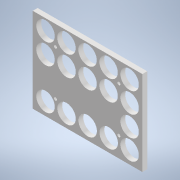
# Autodesk Inventor part: Conectores1
Saved by Autodesk Inventor 2020.3 (Build 243373000, 373)
## iProperties
Created: 2021-04-09
Part Number: Conectores1
Material: Generic
Document SubType Name: Modeling
Designer: juanp
Density: 1 g/cm^3
Appearance: Default
Autodesk Inventor part; units mm, degrees
(part 1 of 8)
ref_plane "YZ Plane" through (0, 0, 0) normal (1, 0, 0) x (0, 1, 0)
ref_plane "XZ Plane" through (0, 0, 0) normal (0, 1, 0) x (-1, 0, 0)
ref_plane "XY Plane" through (0, 0, 0) normal (0, 0, 1) x (1, 0, 0)
sketch "Sketch1" plane through (0, 0, 0) normal (0, 0, 1) x (1, 0, 0)
  arc A0 (61.2864, 36.699) -> (61.2864, 35.945) centre (61.2864, 36.322) ccw
  arc A1 (61.2864, 35.945) -> (61.2864, 36.699) centre (61.2864, 36.322) ccw
  arc A2 (61.2864, 36.699) -> (61.2864, 35.945) centre (61.2864, 36.322) ccw
  arc A3 (61.2864, 35.945) -> (61.2864, 36.699) centre (61.2864, 36.322) ccw
  arc A4 (61.2864, 34.159) -> (61.2864, 33.405) centre (61.2864, 33.782) ccw
  arc A5 (61.2864, 33.405) -> (61.2864, 34.159) centre (61.2864, 33.782) ccw
  arc A6 (61.2864, 34.159) -> (61.2864, 33.405) centre (61.2864, 33.782) ccw
  arc A7 (61.2864, 33.405) -> (61.2864, 34.159) centre (61.2864, 33.782) ccw
  arc A8 (58.7464, 36.699) -> (58.7464, 35.945) centre (58.7464, 36.322) ccw
  arc A9 (58.7464, 35.945) -> (58.7464, 36.699) centre (58.7464, 36.322) ccw
  arc A10 (58.7464, 36.699) -> (58.7464, 35.945) centre (58.7464, 36.322) ccw
  arc A11 (58.7464, 35.945) -> (58.7464, 36.699) centre (58.7464, 36.322) ccw
  arc A12 (58.7464, 34.159) -> (58.7464, 33.405) centre (58.7464, 33.782) ccw
  arc A13 (58.7464, 33.405) -> (58.7464, 34.159) centre (58.7464, 33.782) ccw
  arc A14 (58.7464, 34.159) -> (58.7464, 33.405) centre (58.7464, 33.782) ccw
  arc A15 (58.7464, 33.405) -> (58.7464, 34.159) centre (58.7464, 33.782) ccw
  arc A16 (56.2064, 36.699) -> (56.2064, 35.945) centre (56.2064, 36.322) ccw
  arc A17 (56.2064, 35.945) -> (56.2064, 36.699) centre (56.2064, 36.322) ccw
  arc A18 (56.2064, 36.699) -> (56.2064, 35.945) centre (56.2064, 36.322) ccw
  arc A19 (56.2064, 35.945) -> (56.2064, 36.699) centre (56.2064, 36.322) ccw
  arc A20 (56.2064, 34.159) -> (56.2064, 33.405) centre (56.2064, 33.782) ccw
  arc A21 (56.2064, 33.405) -> (56.2064, 34.159) centre (56.2064, 33.782) ccw
  arc A22 (56.2064, 34.159) -> (56.2064, 33.405) centre (56.2064, 33.782) ccw
  arc A23 (56.2064, 33.405) -> (56.2064, 34.159) centre (56.2064, 33.782) ccw
  arc A24 (53.6664, 36.699) -> (53.6664, 35.945) centre (53.6664, 36.322) ccw
  arc A25 (53.6664, 35.945) -> (53.6664, 36.699) centre (53.6664, 36.322) ccw
  arc A26 (53.6664, 36.699) -> (53.6664, 35.945) centre (53.6664, 36.322) ccw
  arc A27 (53.6664, 35.945) -> (53.6664, 36.699) centre (53.6664, 36.322) ccw
  arc A28 (53.6664, 34.159) -> (53.6664, 33.405) centre (53.6664, 33.782) ccw
  arc A29 (53.6664, 33.405) -> (53.6664, 34.159) centre (53.6664, 33.782) ccw
  arc A30 (53.6664, 34.159) -> (53.6664, 33.405) centre (53.6664, 33.782) ccw
  arc A31 (53.6664, 33.405) -> (53.6664, 34.159) centre (53.6664, 33.782) ccw
  arc A32 (51.1264, 36.699) -> (51.1264, 35.945) centre (51.1264, 36.322) ccw
  arc A33 (51.1264, 35.945) -> (51.1264, 36.699) centre (51.1264, 36.322) ccw
  arc A34 (51.1264, 36.699) -> (51.1264, 35.945) centre (51.1264, 36.322) ccw
  arc A35 (51.1264, 35.945) -> (51.1264, 36.699) centre (51.1264, 36.322) ccw
  arc A36 (51.1264, 34.159) -> (51.1264, 33.405) centre (51.1264, 33.782) ccw
  arc A37 (51.1264, 33.405) -> (51.1264, 34.159) centre (51.1264, 33.782) ccw
  arc A38 (51.1264, 34.159) -> (51.1264, 33.405) centre (51.1264, 33.782) ccw
  arc A39 (51.1264, 33.405) -> (51.1264, 34.159) centre (51.1264, 33.782) ccw
  arc A40 (9.0927, 77.8361) -> (9.0927, 75.8281) centre (9.0927, 76.8321) ccw
  arc A41 (9.0927, 75.8281) -> (9.0927, 77.8361) centre (9.0927, 76.8321) ccw
  arc A42 (9.0927, 77.8361) -> (9.0927, 75.8281) centre (9.0927, 76.8321) ccw
  arc A43 (9.0927, 75.8281) -> (9.0927, 77.8361) centre (9.0927, 76.8321) ccw
  arc A44 (12.0927, 72.8361) -> (12.0927, 70.8281) centre (12.0927, 71.8321) ccw
  arc A45 (12.0927, 70.8281) -> (12.0927, 72.8361) centre (12.0927, 71.8321) ccw
  arc A46 (12.0927, 72.8361) -> (12.0927, 70.8281) centre (12.0927, 71.8321) ccw
  arc A47 (12.0927, 70.8281) -> (12.0927, 72.8361) centre (12.0927, 71.8321) ccw
  arc A48 (15.0927, 77.8361) -> (15.0927, 75.8281) centre (15.0927, 76.8321) ccw
  arc A49 (15.0927, 75.8281) -> (15.0927, 77.8361) centre (15.0927, 76.8321) ccw
  arc A50 (15.0927, 77.8361) -> (15.0927, 75.8281) centre (15.0927, 76.8321) ccw
  arc A51 (15.0927, 75.8281) -> (15.0927, 77.8361) centre (15.0927, 76.8321) ccw
  arc A52 (101.4424, 52.9529) -> (101.4424, 54.9609) centre (101.4424, 53.9569) ccw
  arc A53 (101.4424, 54.9609) -> (101.4424, 52.9529) centre (101.4424, 53.9569) ccw
  arc A54 (101.4424, 52.9529) -> (101.4424, 54.9609) centre (101.4424, 53.9569) ccw
  arc A55 (101.4424, 54.9609) -> (101.4424, 52.9529) centre (101.4424, 53.9569) ccw
  arc A56 (95.4424, 52.9529) -> (95.4424, 54.9609) centre (95.4424, 53.9569) ccw
  arc A57 (95.4424, 54.9609) -> (95.4424, 52.9529) centre (95.4424, 53.9569) ccw
  arc A58 (95.4424, 52.9529) -> (95.4424, 54.9609) centre (95.4424, 53.9569) ccw
  arc A59 (95.4424, 54.9609) -> (95.4424, 52.9529) centre (95.4424, 53.9569) ccw
  line L0 (77.9954, 35.7425) -> (76.9954, 35.7425)
  line L1 (76.9954, 35.7425) -> (76.9954, 34.7425)
  line L2 (76.9954, 34.7425) -> (77.9954, 34.7425)
  line L3 (77.9954, 34.7425) -> (77.9954, 35.7425)
  line L4 (80.01, 36.2331) -> (80.01, 34.2519)
  arc A60 (79.5147, 34.2519) -> (80.5053, 34.2519) centre (80.01, 34.2519) ccw
  arc A61 (80.5053, 36.2331) -> (79.5147, 36.2331) centre (80.01, 36.2331) ccw
  line L5 (80.01, 36.2331) -> (80.01, 34.2519)
  arc A62 (79.5147, 34.2519) -> (80.5053, 34.2519) centre (80.01, 34.2519) ccw
  arc A63 (80.5053, 36.2331) -> (79.5147, 36.2331) centre (80.01, 36.2331) ccw
  line L6 (74.9808, 36.2331) -> (74.9808, 34.2519)
  arc A64 (74.4855, 34.2519) -> (75.4761, 34.2519) centre (74.9808, 34.2519) ccw
  arc A65 (75.4761, 36.2331) -> (74.4855, 36.2331) centre (74.9808, 36.2331) ccw
  line L7 (74.9808, 36.2331) -> (74.9808, 34.2519)
  arc A66 (74.4855, 34.2519) -> (75.4761, 34.2519) centre (74.9808, 34.2519) ccw
  arc A67 (75.4761, 36.2331) -> (74.4855, 36.2331) centre (74.9808, 36.2331) ccw
  arc A68 (35.56, 36.699) -> (35.56, 35.945) centre (35.56, 36.322) ccw
  arc A69 (35.56, 35.945) -> (35.56, 36.699) centre (35.56, 36.322) ccw
  arc A70 (35.56, 36.699) -> (35.56, 35.945) centre (35.56, 36.322) ccw
  arc A71 (35.56, 35.945) -> (35.56, 36.699) centre (35.56, 36.322) ccw
  arc A72 (35.56, 34.159) -> (35.56, 33.405) centre (35.56, 33.782) ccw
  arc A73 (35.56, 33.405) -> (35.56, 34.159) centre (35.56, 33.782) ccw
  arc A74 (35.56, 34.159) -> (35.56, 33.405) centre (35.56, 33.782) ccw
  arc A75 (35.56, 33.405) -> (35.56, 34.159) centre (35.56, 33.782) ccw
  arc A76 (33.02, 36.699) -> (33.02, 35.945) centre (33.02, 36.322) ccw
  arc A77 (33.02, 35.945) -> (33.02, 36.699) centre (33.02, 36.322) ccw
  arc A78 (33.02, 36.699) -> (33.02, 35.945) centre (33.02, 36.322) ccw
  arc A79 (33.02, 35.945) -> (33.02, 36.699) centre (33.02, 36.322) ccw
  arc A80 (33.02, 34.159) -> (33.02, 33.405) centre (33.02, 33.782) ccw
  arc A81 (33.02, 33.405) -> (33.02, 34.159) centre (33.02, 33.782) ccw
  arc A82 (33.02, 34.159) -> (33.02, 33.405) centre (33.02, 33.782) ccw
  arc A83 (33.02, 33.405) -> (33.02, 34.159) centre (33.02, 33.782) ccw
  arc A84 (30.48, 36.699) -> (30.48, 35.945) centre (30.48, 36.322) ccw
  arc A85 (30.48, 35.945) -> (30.48, 36.699) centre (30.48, 36.322) ccw
  arc A86 (30.48, 36.699) -> (30.48, 35.945) centre (30.48, 36.322) ccw
  arc A87 (30.48, 35.945) -> (30.48, 36.699) centre (30.48, 36.322) ccw
  arc A88 (30.48, 34.159) -> (30.48, 33.405) centre (30.48, 33.782) ccw
  arc A89 (30.48, 33.405) -> (30.48, 34.159) centre (30.48, 33.782) ccw
  arc A90 (30.48, 34.159) -> (30.48, 33.405) centre (30.48, 33.782) ccw
  arc A91 (30.48, 33.405) -> (30.48, 34.159) centre (30.48, 33.782) ccw
  arc A92 (27.94, 36.699) -> (27.94, 35.945) centre (27.94, 36.322) ccw
  arc A93 (27.94, 35.945) -> (27.94, 36.699) centre (27.94, 36.322) ccw
  arc A94 (27.94, 36.699) -> (27.94, 35.945) centre (27.94, 36.322) ccw
  arc A95 (27.94, 35.945) -> (27.94, 36.699) centre (27.94, 36.322) ccw
  arc A96 (27.94, 34.159) -> (27.94, 33.405) centre (27.94, 33.782) ccw
  arc A97 (27.94, 33.405) -> (27.94, 34.159) centre (27.94, 33.782) ccw
  arc A98 (27.94, 34.159) -> (27.94, 33.405) centre (27.94, 33.782) ccw
  arc A99 (27.94, 33.405) -> (27.94, 34.159) centre (27.94, 33.782) ccw
  arc A100 (25.4, 36.699) -> (25.4, 35.945) centre (25.4, 36.322) ccw
  arc A101 (25.4, 35.945) -> (25.4, 36.699) centre (25.4, 36.322) ccw
  arc A102 (25.4, 36.699) -> (25.4, 35.945) centre (25.4, 36.322) ccw
  arc A103 (25.4, 35.945) -> (25.4, 36.699) centre (25.4, 36.322) ccw
  arc A104 (25.4, 34.159) -> (25.4, 33.405) centre (25.4, 33.782) ccw
  arc A105 (25.4, 33.405) -> (25.4, 34.159) centre (25.4, 33.782) ccw
  arc A106 (25.4, 34.159) -> (25.4, 33.405) centre (25.4, 33.782) ccw
  arc A107 (25.4, 33.405) -> (25.4, 34.159) centre (25.4, 33.782) ccw
  arc A108 (22.86, 36.699) -> (22.86, 35.945) centre (22.86, 36.322) ccw
  arc A109 (22.86, 35.945) -> (22.86, 36.699) centre (22.86, 36.322) ccw
  arc A110 (22.86, 36.699) -> (22.86, 35.945) centre (22.86, 36.322) ccw
  arc A111 (22.86, 35.945) -> (22.86, 36.699) centre (22.86, 36.322) ccw
  arc A112 (22.86, 34.159) -> (22.86, 33.405) centre (22.86, 33.782) ccw
  arc A113 (22.86, 33.405) -> (22.86, 34.159) centre (22.86, 33.782) ccw
  arc A114 (22.86, 34.159) -> (22.86, 33.405) centre (22.86, 33.782) ccw
  arc A115 (22.86, 33.405) -> (22.86, 34.159) centre (22.86, 33.782) ccw
  arc A116 (20.32, 36.699) -> (20.32, 35.945) centre (20.32, 36.322) ccw
  arc A117 (20.32, 35.945) -> (20.32, 36.699) centre (20.32, 36.322) ccw
  arc A118 (20.32, 36.699) -> (20.32, 35.945) centre (20.32, 36.322) ccw
  arc A119 (20.32, 35.945) -> (20.32, 36.699) centre (20.32, 36.322) ccw
  arc A120 (20.32, 34.159) -> (20.32, 33.405) centre (20.32, 33.782) ccw
  arc A121 (20.32, 33.405) -> (20.32, 34.159) centre (20.32, 33.782) ccw
  arc A122 (20.32, 34.159) -> (20.32, 33.405) centre (20.32, 33.782) ccw
  arc A123 (20.32, 33.405) -> (20.32, 34.159) centre (20.32, 33.782) ccw
  arc A124 (17.78, 36.699) -> (17.78, 35.945) centre (17.78, 36.322) ccw
  arc A125 (17.78, 35.945) -> (17.78, 36.699) centre (17.78, 36.322) ccw
  arc A126 (17.78, 36.699) -> (17.78, 35.945) centre (17.78, 36.322) ccw
  arc A127 (17.78, 35.945) -> (17.78, 36.699) centre (17.78, 36.322) ccw
  arc A128 (17.78, 34.159) -> (17.78, 33.405) centre (17.78, 33.782) ccw
  arc A129 (17.78, 33.405) -> (17.78, 34.159) centre (17.78, 33.782) ccw
  arc A130 (17.78, 34.159) -> (17.78, 33.405) centre (17.78, 33.782) ccw
  arc A131 (17.78, 33.405) -> (17.78, 34.159) centre (17.78, 33.782) ccw
  arc A132 (15.24, 36.699) -> (15.24, 35.945) centre (15.24, 36.322) ccw
  arc A133 (15.24, 35.945) -> (15.24, 36.699) centre (15.24, 36.322) ccw
  arc A134 (15.24, 36.699) -> (15.24, 35.945) centre (15.24, 36.322) ccw
  arc A135 (15.24, 35.945) -> (15.24, 36.699) centre (15.24, 36.322) ccw
  arc A136 (15.24, 34.159) -> (15.24, 33.405) centre (15.24, 33.782) ccw
  arc A137 (15.24, 33.405) -> (15.24, 34.159) centre (15.24, 33.782) ccw
  arc A138 (15.24, 34.159) -> (15.24, 33.405) centre (15.24, 33.782) ccw
  arc A139 (15.24, 33.405) -> (15.24, 34.159) centre (15.24, 33.782) ccw
  arc A140 (12.7, 36.699) -> (12.7, 35.945) centre (12.7, 36.322) ccw
  arc A141 (12.7, 35.945) -> (12.7, 36.699) centre (12.7, 36.322) ccw
  arc A142 (12.7, 36.699) -> (12.7, 35.945) centre (12.7, 36.322) ccw
  arc A143 (12.7, 35.945) -> (12.7, 36.699) centre (12.7, 36.322) ccw
  arc A144 (12.7, 34.159) -> (12.7, 33.405) centre (12.7, 33.782) ccw
  arc A145 (12.7, 33.405) -> (12.7, 34.159) centre (12.7, 33.782) ccw
  arc A146 (12.7, 34.159) -> (12.7, 33.405) centre (12.7, 33.782) ccw
  arc A147 (12.7, 33.405) -> (12.7, 34.159) centre (12.7, 33.782) ccw
  arc A148 (10.16, 36.699) -> (10.16, 35.945) centre (10.16, 36.322) ccw
  arc A149 (10.16, 35.945) -> (10.16, 36.699) centre (10.16, 36.322) ccw
  arc A150 (10.16, 36.699) -> (10.16, 35.945) centre (10.16, 36.322) ccw
  arc A151 (10.16, 35.945) -> (10.16, 36.699) centre (10.16, 36.322) ccw
  arc A152 (10.16, 34.159) -> (10.16, 33.405) centre (10.16, 33.782) ccw
  arc A153 (10.16, 33.405) -> (10.16, 34.159) centre (10.16, 33.782) ccw
  arc A154 (10.16, 34.159) -> (10.16, 33.405) centre (10.16, 33.782) ccw
  arc A155 (10.16, 33.405) -> (10.16, 34.159) centre (10.16, 33.782) ccw
  arc A156 (7.62, 36.699) -> (7.62, 35.945) centre (7.62, 36.322) ccw
  arc A157 (7.62, 35.945) -> (7.62, 36.699) centre (7.62, 36.322) ccw
  arc A158 (7.62, 36.699) -> (7.62, 35.945) centre (7.62, 36.322) ccw
  arc A159 (7.62, 35.945) -> (7.62, 36.699) centre (7.62, 36.322) ccw
  arc A160 (7.62, 34.159) -> (7.62, 33.405) centre (7.62, 33.782) ccw
  arc A161 (7.62, 33.405) -> (7.62, 34.159) centre (7.62, 33.782) ccw
  arc A162 (7.62, 34.159) -> (7.62, 33.405) centre (7.62, 33.782) ccw
  arc A163 (7.62, 33.405) -> (7.62, 34.159) centre (7.62, 33.782) ccw
  arc A164 (74.3504, 57.4609) -> (74.3504, 55.4529) centre (74.3504, 56.4569) ccw
  arc A165 (74.3504, 55.4529) -> (74.3504, 57.4609) centre (74.3504, 56.4569) ccw
  arc A166 (74.3504, 57.4609) -> (74.3504, 55.4529) centre (74.3504, 56.4569) ccw
  arc A167 (74.3504, 55.4529) -> (74.3504, 57.4609) centre (74.3504, 56.4569) ccw
  arc A168 (74.3504, 52.4609) -> (74.3504, 50.4529) centre (74.3504, 51.4569) ccw
  arc A169 (74.3504, 50.4529) -> (74.3504, 52.4609) centre (74.3504, 51.4569) ccw
  arc A170 (74.3504, 52.4609) -> (74.3504, 50.4529) centre (74.3504, 51.4569) ccw
  arc A171 (74.3504, 50.4529) -> (74.3504, 52.4609) centre (74.3504, 51.4569) ccw
  arc A172 (79.3504, 52.4609) -> (79.3504, 50.4529) centre (79.3504, 51.4569) ccw
  arc A173 (79.3504, 50.4529) -> (79.3504, 52.4609) centre (79.3504, 51.4569) ccw
  arc A174 (79.3504, 52.4609) -> (79.3504, 50.4529) centre (79.3504, 51.4569) ccw
  arc A175 (79.3504, 50.4529) -> (79.3504, 52.4609) centre (79.3504, 51.4569) ccw
  arc A176 (79.3504, 57.4609) -> (79.3504, 55.4529) centre (79.3504, 56.4569) ccw
  arc A177 (79.3504, 55.4529) -> (79.3504, 57.4609) centre (79.3504, 56.4569) ccw
  arc A178 (79.3504, 57.4609) -> (79.3504, 55.4529) centre (79.3504, 56.4569) ccw
  arc A179 (79.3504, 55.4529) -> (79.3504, 57.4609) centre (79.3504, 56.4569) ccw
  line L8 (23.36, 25.392) -> (22.36, 25.392)
  line L9 (22.36, 25.392) -> (22.36, 24.392)
  line L10 (22.36, 24.392) -> (23.36, 24.392)
  line L11 (23.36, 24.392) -> (23.36, 25.392)
  line L12 (23.36, 26.408) -> (22.36, 26.408)
  line L13 (22.36, 26.408) -> (22.36, 25.408)
  line L14 (22.36, 25.408) -> (23.36, 25.408)
  line L15 (23.36, 25.408) -> (23.36, 26.408)
  line L16 (20.82, 25.392) -> (19.82, 25.392)
  line L17 (19.82, 25.392) -> (19.82, 24.392)
  line L18 (19.82, 24.392) -> (20.82, 24.392)
  line L19 (20.82, 24.392) -> (20.82, 25.392)
  line L20 (20.82, 26.408) -> (19.82, 26.408)
  line L21 (19.82, 26.408) -> (19.82, 25.408)
  line L22 (19.82, 25.408) -> (20.82, 25.408)
  line L23 (20.82, 25.408) -> (20.82, 26.408)
  line L24 (18.28, 25.392) -> (17.28, 25.392)
  line L25 (17.28, 25.392) -> (17.28, 24.392)
  line L26 (17.28, 24.392) -> (18.28, 24.392)
  line L27 (18.28, 24.392) -> (18.28, 25.392)
  line L28 (18.28, 26.408) -> (17.28, 26.408)
  line L29 (17.28, 26.408) -> (17.28, 25.408)
  line L30 (17.28, 25.408) -> (18.28, 25.408)
  line L31 (18.28, 25.408) -> (18.28, 26.408)
  line L32 (15.74, 25.392) -> (14.74, 25.392)
  line L33 (14.74, 25.392) -> (14.74, 24.392)
  line L34 (14.74, 24.392) -> (15.74, 24.392)
  line L35 (15.74, 24.392) -> (15.74, 25.392)
  line L36 (15.74, 26.408) -> (14.74, 26.408)
  line L37 (14.74, 26.408) -> (14.74, 25.408)
  line L38 (14.74, 25.408) -> (15.74, 25.408)
  line L39 (15.74, 25.408) -> (15.74, 26.408)
  line L40 (13.2, 25.392) -> (12.2, 25.392)
  line L41 (12.2, 25.392) -> (12.2, 24.392)
  line L42 (12.2, 24.392) -> (13.2, 24.392)
  line L43 (13.2, 24.392) -> (13.2, 25.392)
  line L44 (13.2, 26.408) -> (12.2, 26.408)
  line L45 (12.2, 26.408) -> (12.2, 25.408)
  line L46 (12.2, 25.408) -> (13.2, 25.408)
  line L47 (13.2, 25.408) -> (13.2, 26.408)
  line L48 (10.66, 25.392) -> (9.66, 25.392)
  line L49 (9.66, 25.392) -> (9.66, 24.392)
  line L50 (9.66, 24.392) -> (10.66, 24.392)
  line L51 (10.66, 24.392) -> (10.66, 25.392)
  line L52 (10.66, 26.408) -> (9.66, 26.408)
  line L53 (9.66, 26.408) -> (9.66, 25.408)
  line L54 (9.66, 25.408) -> (10.66, 25.408)
  line L55 (10.66, 25.408) -> (10.66, 26.408)
  line L56 (8.12, 25.392) -> (7.12, 25.392)
  line L57 (7.12, 25.392) -> (7.12, 24.392)
  line L58 (7.12, 24.392) -> (8.12, 24.392)
  line L59 (8.12, 24.392) -> (8.12, 25.392)
  line L60 (8.12, 26.408) -> (7.12, 26.408)
  line L61 (7.12, 26.408) -> (7.12, 25.408)
  line L62 (7.12, 25.408) -> (8.12, 25.408)
  line L63 (8.12, 25.408) -> (8.12, 26.408)
  line L64 (22.86, 26.0604) -> (22.86, 24.7396)
  arc A180 (22.5298, 24.7396) -> (23.1902, 24.7396) centre (22.86, 24.7396) ccw
  arc A181 (23.1902, 26.0604) -> (22.5298, 26.0604) centre (22.86, 26.0604) ccw
  line L65 (22.86, 26.0604) -> (22.86, 24.7396)
  arc A182 (22.5298, 24.7396) -> (23.1902, 24.7396) centre (22.86, 24.7396) ccw
  arc A183 (23.1902, 26.0604) -> (22.5298, 26.0604) centre (22.86, 26.0604) ccw
  line L66 (20.32, 26.0604) -> (20.32, 24.7396)
  arc A184 (19.9898, 24.7396) -> (20.6502, 24.7396) centre (20.32, 24.7396) ccw
  arc A185 (20.6502, 26.0604) -> (19.9898, 26.0604) centre (20.32, 26.0604) ccw
  line L67 (20.32, 26.0604) -> (20.32, 24.7396)
  arc A186 (19.9898, 24.7396) -> (20.6502, 24.7396) centre (20.32, 24.7396) ccw
  arc A187 (20.6502, 26.0604) -> (19.9898, 26.0604) centre (20.32, 26.0604) ccw
  line L68 (17.78, 26.0604) -> (17.78, 24.7396)
  arc A188 (17.4498, 24.7396) -> (18.1102, 24.7396) centre (17.78, 24.7396) ccw
  arc A189 (18.1102, 26.0604) -> (17.4498, 26.0604) centre (17.78, 26.0604) ccw
  line L69 (17.78, 26.0604) -> (17.78, 24.7396)
  arc A190 (17.4498, 24.7396) -> (18.1102, 24.7396) centre (17.78, 24.7396) ccw
  arc A191 (18.1102, 26.0604) -> (17.4498, 26.0604) centre (17.78, 26.0604) ccw
  line L70 (15.24, 26.0604) -> (15.24, 24.7396)
  arc A192 (14.9098, 24.7396) -> (15.5702, 24.7396) centre (15.24, 24.7396) ccw
  arc A193 (15.5702, 26.0604) -> (14.9098, 26.0604) centre (15.24, 26.0604) ccw
  line L71 (15.24, 26.0604) -> (15.24, 24.7396)
  arc A194 (14.9098, 24.7396) -> (15.5702, 24.7396) centre (15.24, 24.7396) ccw
  arc A195 (15.5702, 26.0604) -> (14.9098, 26.0604) centre (15.24, 26.0604) ccw
  line L72 (12.7, 26.0604) -> (12.7, 24.7396)
  arc A196 (12.3698, 24.7396) -> (13.0302, 24.7396) centre (12.7, 24.7396) ccw
  arc A197 (13.0302, 26.0604) -> (12.3698, 26.0604) centre (12.7, 26.0604) ccw
  line L73 (12.7, 26.0604) -> (12.7, 24.7396)
  arc A198 (12.3698, 24.7396) -> (13.0302, 24.7396) centre (12.7, 24.7396) ccw
  arc A199 (13.0302, 26.0604) -> (12.3698, 26.0604) centre (12.7, 26.0604) ccw
  line L74 (10.16, 26.0604) -> (10.16, 24.7396)
  arc A200 (9.8298, 24.7396) -> (10.4902, 24.7396) centre (10.16, 24.7396) ccw
  arc A201 (10.4902, 26.0604) -> (9.8298, 26.0604) centre (10.16, 26.0604) ccw
  line L75 (10.16, 26.0604) -> (10.16, 24.7396)
  arc A202 (9.8298, 24.7396) -> (10.4902, 24.7396) centre (10.16, 24.7396) ccw
  arc A203 (10.4902, 26.0604) -> (9.8298, 26.0604) centre (10.16, 26.0604) ccw
  line L76 (7.62, 26.0604) -> (7.62, 24.7396)
  arc A204 (7.2898, 24.7396) -> (7.9502, 24.7396) centre (7.62, 24.7396) ccw
  arc A205 (7.9502, 26.0604) -> (7.2898, 26.0604) centre (7.62, 26.0604) ccw
  line L77 (7.62, 26.0604) -> (7.62, 24.7396)
  arc A206 (7.2898, 24.7396) -> (7.9502, 24.7396) centre (7.62, 24.7396) ccw
  arc A207 (7.9502, 26.0604) -> (7.2898, 26.0604) centre (7.62, 26.0604) ccw
  line L78 (45.601, 25.408) -> (46.601, 25.408)
  line L79 (46.601, 25.408) -> (46.601, 26.408)
  line L80 (46.601, 26.408) -> (45.601, 26.408)
  line L81 (45.601, 26.408) -> (45.601, 25.408)
  line L82 (45.601, 24.392) -> (46.601, 24.392)
  line L83 (46.601, 24.392) -> (46.601, 25.392)
  line L84 (46.601, 25.392) -> (45.601, 25.392)
  line L85 (45.601, 25.392) -> (45.601, 24.392)
  line L86 (48.141, 25.408) -> (49.141, 25.408)
  line L87 (49.141, 25.408) -> (49.141, 26.408)
  line L88 (49.141, 26.408) -> (48.141, 26.408)
  line L89 (48.141, 26.408) -> (48.141, 25.408)
  line L90 (48.141, 24.392) -> (49.141, 24.392)
  line L91 (49.141, 24.392) -> (49.141, 25.392)
  line L92 (49.141, 25.392) -> (48.141, 25.392)
  line L93 (48.141, 25.392) -> (48.141, 24.392)
  line L94 (50.681, 25.408) -> (51.681, 25.408)
  line L95 (51.681, 25.408) -> (51.681, 26.408)
  line L96 (51.681, 26.408) -> (50.681, 26.408)
  line L97 (50.681, 26.408) -> (50.681, 25.408)
  line L98 (50.681, 24.392) -> (51.681, 24.392)
  line L99 (51.681, 24.392) -> (51.681, 25.392)
  line L100 (51.681, 25.392) -> (50.681, 25.392)
  line L101 (50.681, 25.392) -> (50.681, 24.392)
  line L102 (53.221, 25.408) -> (54.221, 25.408)
  line L103 (54.221, 25.408) -> (54.221, 26.408)
  line L104 (54.221, 26.408) -> (53.221, 26.408)
  line L105 (53.221, 26.408) -> (53.221, 25.408)
  line L106 (53.221, 24.392) -> (54.221, 24.392)
  line L107 (54.221, 24.392) -> (54.221, 25.392)
  line L108 (54.221, 25.392) -> (53.221, 25.392)
  line L109 (53.221, 25.392) -> (53.221, 24.392)
  line L110 (55.761, 25.408) -> (56.761, 25.408)
  line L111 (56.761, 25.408) -> (56.761, 26.408)
  line L112 (56.761, 26.408) -> (55.761, 26.408)
  line L113 (55.761, 26.408) -> (55.761, 25.408)
  line L114 (55.761, 24.392) -> (56.761, 24.392)
  line L115 (56.761, 24.392) -> (56.761, 25.392)
  line L116 (56.761, 25.392) -> (55.761, 25.392)
  line L117 (55.761, 25.392) -> (55.761, 24.392)
  line L118 (46.101, 24.7396) -> (46.101, 26.0604)
  arc A208 (46.4312, 26.0604) -> (45.7708, 26.0604) centre (46.101, 26.0604) ccw
  arc A209 (45.7708, 24.7396) -> (46.4312, 24.7396) centre (46.101, 24.7396) ccw
  line L119 (46.101, 24.7396) -> (46.101, 26.0604)
  arc A210 (46.4312, 26.0604) -> (45.7708, 26.0604) centre (46.101, 26.0604) ccw
  arc A211 (45.7708, 24.7396) -> (46.4312, 24.7396) centre (46.101, 24.7396) ccw
  line L120 (48.641, 24.7396) -> (48.641, 26.0604)
  arc A212 (48.9712, 26.0604) -> (48.3108, 26.0604) centre (48.641, 26.0604) ccw
  arc A213 (48.3108, 24.7396) -> (48.9712, 24.7396) centre (48.641, 24.7396) ccw
  line L121 (48.641, 24.7396) -> (48.641, 26.0604)
  arc A214 (48.9712, 26.0604) -> (48.3108, 26.0604) centre (48.641, 26.0604) ccw
  arc A215 (48.3108, 24.7396) -> (48.9712, 24.7396) centre (48.641, 24.7396) ccw
  line L122 (51.181, 24.7396) -> (51.181, 26.0604)
  arc A216 (51.5112, 26.0604) -> (50.8508, 26.0604) centre (51.181, 26.0604) ccw
  arc A217 (50.8508, 24.7396) -> (51.5112, 24.7396) centre (51.181, 24.7396) ccw
  line L123 (51.181, 24.7396) -> (51.181, 26.0604)
  arc A218 (51.5112, 26.0604) -> (50.8508, 26.0604) centre (51.181, 26.0604) ccw
  arc A219 (50.8508, 24.7396) -> (51.5112, 24.7396) centre (51.181, 24.7396) ccw
  line L124 (53.721, 24.7396) -> (53.721, 26.0604)
  arc A220 (54.0512, 26.0604) -> (53.3908, 26.0604) centre (53.721, 26.0604) ccw
  arc A221 (53.3908, 24.7396) -> (54.0512, 24.7396) centre (53.721, 24.7396) ccw
  line L125 (53.721, 24.7396) -> (53.721, 26.0604)
  arc A222 (54.0512, 26.0604) -> (53.3908, 26.0604) centre (53.721, 26.0604) ccw
  arc A223 (53.3908, 24.7396) -> (54.0512, 24.7396) centre (53.721, 24.7396) ccw
  line L126 (56.261, 24.7396) -> (56.261, 26.0604)
  arc A224 (56.5912, 26.0604) -> (55.9308, 26.0604) centre (56.261, 26.0604) ccw
  arc A225 (55.9308, 24.7396) -> (56.5912, 24.7396) centre (56.261, 24.7396) ccw
  line L127 (56.261, 24.7396) -> (56.261, 26.0604)
  arc A226 (56.5912, 26.0604) -> (55.9308, 26.0604) centre (56.261, 26.0604) ccw
  arc A227 (55.9308, 24.7396) -> (56.5912, 24.7396) centre (56.261, 24.7396) ccw
  arc A228 (52.2831, 56.8811) -> (52.2831, 54.8731) centre (52.2831, 55.8771) ccw
  arc A229 (52.2831, 54.8731) -> (52.2831, 56.8811) centre (52.2831, 55.8771) ccw
  arc A230 (52.2831, 56.8811) -> (52.2831, 54.8731) centre (52.2831, 55.8771) ccw
  arc A231 (52.2831, 54.8731) -> (52.2831, 56.8811) centre (52.2831, 55.8771) ccw
  arc A232 (55.2831, 51.8811) -> (55.2831, 49.8731) centre (55.2831, 50.8771) ccw
  arc A233 (55.2831, 49.8731) -> (55.2831, 51.8811) centre (55.2831, 50.8771) ccw
  arc A234 (55.2831, 51.8811) -> (55.2831, 49.8731) centre (55.2831, 50.8771) ccw
  arc A235 (55.2831, 49.8731) -> (55.2831, 51.8811) centre (55.2831, 50.8771) ccw
  arc A236 (58.2831, 56.8811) -> (58.2831, 54.8731) centre (58.2831, 55.8771) ccw
  arc A237 (58.2831, 54.8731) -> (58.2831, 56.8811) centre (58.2831, 55.8771) ccw
  arc A238 (58.2831, 56.8811) -> (58.2831, 54.8731) centre (58.2831, 55.8771) ccw
  arc A239 (58.2831, 54.8731) -> (58.2831, 56.8811) centre (58.2831, 55.8771) ccw
  arc A240 (52.2196, 78.0102) -> (52.2196, 76.0022) centre (52.2196, 77.0062) ccw
  arc A241 (52.2196, 76.0022) -> (52.2196, 78.0102) centre (52.2196, 77.0062) ccw
  arc A242 (52.2196, 78.0102) -> (52.2196, 76.0022) centre (52.2196, 77.0062) ccw
  arc A243 (52.2196, 76.0022) -> (52.2196, 78.0102) centre (52.2196, 77.0062) ccw
  arc A244 (55.2196, 73.0102) -> (55.2196, 71.0022) centre (55.2196, 72.0062) ccw
  arc A245 (55.2196, 71.0022) -> (55.2196, 73.0102) centre (55.2196, 72.0062) ccw
  arc A246 (55.2196, 73.0102) -> (55.2196, 71.0022) centre (55.2196, 72.0062) ccw
  arc A247 (55.2196, 71.0022) -> (55.2196, 73.0102) centre (55.2196, 72.0062) ccw
  arc A248 (58.2196, 78.0102) -> (58.2196, 76.0022) centre (58.2196, 77.0062) ccw
  arc A249 (58.2196, 76.0022) -> (58.2196, 78.0102) centre (58.2196, 77.0062) ccw
  arc A250 (58.2196, 78.0102) -> (58.2196, 76.0022) centre (58.2196, 77.0062) ccw
  arc A251 (58.2196, 76.0022) -> (58.2196, 78.0102) centre (58.2196, 77.0062) ccw
  arc A252 (95.4424, 13.1452) -> (95.4424, 11.1372) centre (95.4424, 12.1412) ccw
  arc A253 (95.4424, 11.1372) -> (95.4424, 13.1452) centre (95.4424, 12.1412) ccw
  arc A254 (95.4424, 13.1452) -> (95.4424, 11.1372) centre (95.4424, 12.1412) ccw
  arc A255 (95.4424, 11.1372) -> (95.4424, 13.1452) centre (95.4424, 12.1412) ccw
  arc A256 (101.4424, 13.1452) -> (101.4424, 11.1372) centre (101.4424, 12.1412) ccw
  arc A257 (101.4424, 11.1372) -> (101.4424, 13.1452) centre (101.4424, 12.1412) ccw
  arc A258 (101.4424, 13.1452) -> (101.4424, 11.1372) centre (101.4424, 12.1412) ccw
  arc A259 (101.4424, 11.1372) -> (101.4424, 13.1452) centre (101.4424, 12.1412) ccw
  arc A260 (95.4358, 33.7936) -> (95.4358, 31.7856) centre (95.4358, 32.7896) ccw
  arc A261 (95.4358, 31.7856) -> (95.4358, 33.7936) centre (95.4358, 32.7896) ccw
  arc A262 (95.4358, 33.7936) -> (95.4358, 31.7856) centre (95.4358, 32.7896) ccw
  arc A263 (95.4358, 31.7856) -> (95.4358, 33.7936) centre (95.4358, 32.7896) ccw
  arc A264 (101.4358, 33.7936) -> (101.4358, 31.7856) centre (101.4358, 32.7896) ccw
  arc A265 (101.4358, 31.7856) -> (101.4358, 33.7936) centre (101.4358, 32.7896) ccw
  arc A266 (101.4358, 33.7936) -> (101.4358, 31.7856) centre (101.4358, 32.7896) ccw
  arc A267 (101.4358, 31.7856) -> (101.4358, 33.7936) centre (101.4358, 32.7896) ccw
  arc A268 (73.8576, 75.8361) -> (73.8576, 73.8281) centre (73.8576, 74.8321) ccw
  arc A269 (73.8576, 73.8281) -> (73.8576, 75.8361) centre (73.8576, 74.8321) ccw
  arc A270 (73.8576, 75.8361) -> (73.8576, 73.8281) centre (73.8576, 74.8321) ccw
  arc A271 (73.8576, 73.8281) -> (73.8576, 75.8361) centre (73.8576, 74.8321) ccw
  arc A272 (79.8576, 75.8361) -> (79.8576, 73.8281) centre (79.8576, 74.8321) ccw
  arc A273 (79.8576, 73.8281) -> (79.8576, 75.8361) centre (79.8576, 74.8321) ccw
  arc A274 (79.8576, 75.8361) -> (79.8576, 73.8281) centre (79.8576, 74.8321) ccw
  arc A275 (79.8576, 73.8281) -> (79.8576, 75.8361) centre (79.8576, 74.8321) ccw
  arc A276 (95.4424, 75.8361) -> (95.4424, 73.8281) centre (95.4424, 74.8321) ccw
  arc A277 (95.4424, 73.8281) -> (95.4424, 75.8361) centre (95.4424, 74.8321) ccw
  arc A278 (95.4424, 75.8361) -> (95.4424, 73.8281) centre (95.4424, 74.8321) ccw
  arc A279 (95.4424, 73.8281) -> (95.4424, 75.8361) centre (95.4424, 74.8321) ccw
  arc A280 (101.4424, 75.8361) -> (101.4424, 73.8281) centre (101.4424, 74.8321) ccw
  arc A281 (101.4424, 73.8281) -> (101.4424, 75.8361) centre (101.4424, 74.8321) ccw
  arc A282 (101.4424, 75.8361) -> (101.4424, 73.8281) centre (101.4424, 74.8321) ccw
  arc A283 (101.4424, 73.8281) -> (101.4424, 75.8361) centre (101.4424, 74.8321) ccw
  arc A284 (36.6796, 9.0846) -> (36.6796, 11.0926) centre (36.6796, 10.0886) ccw
  arc A285 (36.6796, 11.0926) -> (36.6796, 9.0846) centre (36.6796, 10.0886) ccw
  arc A286 (36.6796, 9.0846) -> (36.6796, 11.0926) centre (36.6796, 10.0886) ccw
  arc A287 (36.6796, 11.0926) -> (36.6796, 9.0846) centre (36.6796, 10.0886) ccw
  arc A288 (33.6796, 14.0846) -> (33.6796, 16.0926) centre (33.6796, 15.0886) ccw
  arc A289 (33.6796, 16.0926) -> (33.6796, 14.0846) centre (33.6796, 15.0886) ccw
  arc A290 (33.6796, 14.0846) -> (33.6796, 16.0926) centre (33.6796, 15.0886) ccw
  arc A291 (33.6796, 16.0926) -> (33.6796, 14.0846) centre (33.6796, 15.0886) ccw
  arc A292 (30.6796, 9.0846) -> (30.6796, 11.0926) centre (30.6796, 10.0886) ccw
  arc A293 (30.6796, 11.0926) -> (30.6796, 9.0846) centre (30.6796, 10.0886) ccw
  arc A294 (30.6796, 9.0846) -> (30.6796, 11.0926) centre (30.6796, 10.0886) ccw
  arc A295 (30.6796, 11.0926) -> (30.6796, 9.0846) centre (30.6796, 10.0886) ccw
  arc A296 (31.1842, 57.4609) -> (31.1842, 55.4529) centre (31.1842, 56.4569) ccw
  arc A297 (31.1842, 55.4529) -> (31.1842, 57.4609) centre (31.1842, 56.4569) ccw
  arc A298 (31.1842, 57.4609) -> (31.1842, 55.4529) centre (31.1842, 56.4569) ccw
  arc A299 (31.1842, 55.4529) -> (31.1842, 57.4609) centre (31.1842, 56.4569) ccw
  arc A300 (31.1842, 52.4609) -> (31.1842, 50.4529) centre (31.1842, 51.4569) ccw
  arc A301 (31.1842, 50.4529) -> (31.1842, 52.4609) centre (31.1842, 51.4569) ccw
  arc A302 (31.1842, 52.4609) -> (31.1842, 50.4529) centre (31.1842, 51.4569) ccw
  arc A303 (31.1842, 50.4529) -> (31.1842, 52.4609) centre (31.1842, 51.4569) ccw
  arc A304 (36.1842, 52.4609) -> (36.1842, 50.4529) centre (36.1842, 51.4569) ccw
  arc A305 (36.1842, 50.4529) -> (36.1842, 52.4609) centre (36.1842, 51.4569) ccw
  arc A306 (36.1842, 52.4609) -> (36.1842, 50.4529) centre (36.1842, 51.4569) ccw
  arc A307 (36.1842, 50.4529) -> (36.1842, 52.4609) centre (36.1842, 51.4569) ccw
  arc A308 (36.1842, 57.4609) -> (36.1842, 55.4529) centre (36.1842, 56.4569) ccw
  arc A309 (36.1842, 55.4529) -> (36.1842, 57.4609) centre (36.1842, 56.4569) ccw
  arc A310 (36.1842, 57.4609) -> (36.1842, 55.4529) centre (36.1842, 56.4569) ccw
  arc A311 (36.1842, 55.4529) -> (36.1842, 57.4609) centre (36.1842, 56.4569) ccw
  arc A312 (9.0477, 56.8012) -> (9.0477, 54.7932) centre (9.0477, 55.7972) ccw
  arc A313 (9.0477, 54.7932) -> (9.0477, 56.8012) centre (9.0477, 55.7972) ccw
  arc A314 (9.0477, 56.8012) -> (9.0477, 54.7932) centre (9.0477, 55.7972) ccw
  arc A315 (9.0477, 54.7932) -> (9.0477, 56.8012) centre (9.0477, 55.7972) ccw
  arc A316 (12.0477, 51.8012) -> (12.0477, 49.7932) centre (12.0477, 50.7972) ccw
  arc A317 (12.0477, 49.7932) -> (12.0477, 51.8012) centre (12.0477, 50.7972) ccw
  arc A318 (12.0477, 51.8012) -> (12.0477, 49.7932) centre (12.0477, 50.7972) ccw
  arc A319 (12.0477, 49.7932) -> (12.0477, 51.8012) centre (12.0477, 50.7972) ccw
  arc A320 (15.0477, 56.8012) -> (15.0477, 54.7932) centre (15.0477, 55.7972) ccw
  arc A321 (15.0477, 54.7932) -> (15.0477, 56.8012) centre (15.0477, 55.7972) ccw
  arc A322 (15.0477, 56.8012) -> (15.0477, 54.7932) centre (15.0477, 55.7972) ccw
  arc A323 (15.0477, 54.7932) -> (15.0477, 56.8012) centre (15.0477, 55.7972) ccw
  arc A324 (15.085, 9.0429) -> (15.085, 11.0509) centre (15.085, 10.0469) ccw
  arc A325 (15.085, 11.0509) -> (15.085, 9.0429) centre (15.085, 10.0469) ccw
  arc A326 (15.085, 9.0429) -> (15.085, 11.0509) centre (15.085, 10.0469) ccw
  arc A327 (15.085, 11.0509) -> (15.085, 9.0429) centre (15.085, 10.0469) ccw
  arc A328 (12.085, 14.0429) -> (12.085, 16.0509) centre (12.085, 15.0469) ccw
  arc A329 (12.085, 16.0509) -> (12.085, 14.0429) centre (12.085, 15.0469) ccw
  arc A330 (12.085, 14.0429) -> (12.085, 16.0509) centre (12.085, 15.0469) ccw
  arc A331 (12.085, 16.0509) -> (12.085, 14.0429) centre (12.085, 15.0469) ccw
  arc A332 (9.085, 9.0429) -> (9.085, 11.0509) centre (9.085, 10.0469) ccw
  arc A333 (9.085, 11.0509) -> (9.085, 9.0429) centre (9.085, 10.0469) ccw
  arc A334 (9.085, 9.0429) -> (9.085, 11.0509) centre (9.085, 10.0469) ccw
  arc A335 (9.085, 11.0509) -> (9.085, 9.0429) centre (9.085, 10.0469) ccw
  arc A336 (57.8493, 8.6372) -> (57.8493, 10.6452) centre (57.8493, 9.6412) ccw
  arc A337 (57.8493, 10.6452) -> (57.8493, 8.6372) centre (57.8493, 9.6412) ccw
  arc A338 (57.8493, 8.6372) -> (57.8493, 10.6452) centre (57.8493, 9.6412) ccw
  arc A339 (57.8493, 10.6452) -> (57.8493, 8.6372) centre (57.8493, 9.6412) ccw
  arc A340 (57.8493, 13.6372) -> (57.8493, 15.6452) centre (57.8493, 14.6412) ccw
  arc A341 (57.8493, 15.6452) -> (57.8493, 13.6372) centre (57.8493, 14.6412) ccw
  arc A342 (57.8493, 13.6372) -> (57.8493, 15.6452) centre (57.8493, 14.6412) ccw
  arc A343 (57.8493, 15.6452) -> (57.8493, 13.6372) centre (57.8493, 14.6412) ccw
  arc A344 (52.8493, 13.6372) -> (52.8493, 15.6452) centre (52.8493, 14.6412) ccw
  arc A345 (52.8493, 15.6452) -> (52.8493, 13.6372) centre (52.8493, 14.6412) ccw
  arc A346 (52.8493, 13.6372) -> (52.8493, 15.6452) centre (52.8493, 14.6412) ccw
  arc A347 (52.8493, 15.6452) -> (52.8493, 13.6372) centre (52.8493, 14.6412) ccw
  arc A348 (52.8493, 8.6372) -> (52.8493, 10.6452) centre (52.8493, 9.6412) ccw
  arc A349 (52.8493, 10.6452) -> (52.8493, 8.6372) centre (52.8493, 9.6412) ccw
  arc A350 (52.8493, 8.6372) -> (52.8493, 10.6452) centre (52.8493, 9.6412) ccw
  arc A351 (52.8493, 10.6452) -> (52.8493, 8.6372) centre (52.8493, 9.6412) ccw
  arc A352 (31.0609, 78.4159) -> (31.0609, 76.4079) centre (31.0609, 77.4119) ccw
  arc A353 (31.0609, 76.4079) -> (31.0609, 78.4159) centre (31.0609, 77.4119) ccw
  arc A354 (31.0609, 78.4159) -> (31.0609, 76.4079) centre (31.0609, 77.4119) ccw
  arc A355 (31.0609, 76.4079) -> (31.0609, 78.4159) centre (31.0609, 77.4119) ccw
  arc A356 (31.0609, 73.4159) -> (31.0609, 71.4079) centre (31.0609, 72.4119) ccw
  arc A357 (31.0609, 71.4079) -> (31.0609, 73.4159) centre (31.0609, 72.4119) ccw
  arc A358 (31.0609, 73.4159) -> (31.0609, 71.4079) centre (31.0609, 72.4119) ccw
  arc A359 (31.0609, 71.4079) -> (31.0609, 73.4159) centre (31.0609, 72.4119) ccw
  arc A360 (36.0609, 73.4159) -> (36.0609, 71.4079) centre (36.0609, 72.4119) ccw
  arc A361 (36.0609, 71.4079) -> (36.0609, 73.4159) centre (36.0609, 72.4119) ccw
  arc A362 (36.0609, 73.4159) -> (36.0609, 71.4079) centre (36.0609, 72.4119) ccw
  arc A363 (36.0609, 71.4079) -> (36.0609, 73.4159) centre (36.0609, 72.4119) ccw
  arc A364 (36.0609, 78.4159) -> (36.0609, 76.4079) centre (36.0609, 77.4119) ccw
  arc A365 (36.0609, 76.4079) -> (36.0609, 78.4159) centre (36.0609, 77.4119) ccw
  arc A366 (36.0609, 78.4159) -> (36.0609, 76.4079) centre (36.0609, 77.4119) ccw
  arc A367 (36.0609, 76.4079) -> (36.0609, 78.4159) centre (36.0609, 77.4119) ccw
  arc A368 (79.442, 8.6372) -> (79.442, 10.6452) centre (79.442, 9.6412) ccw
  arc A369 (79.442, 10.6452) -> (79.442, 8.6372) centre (79.442, 9.6412) ccw
  arc A370 (79.442, 8.6372) -> (79.442, 10.6452) centre (79.442, 9.6412) ccw
  arc A371 (79.442, 10.6452) -> (79.442, 8.6372) centre (79.442, 9.6412) ccw
  arc A372 (79.442, 13.6372) -> (79.442, 15.6452) centre (79.442, 14.6412) ccw
  arc A373 (79.442, 15.6452) -> (79.442, 13.6372) centre (79.442, 14.6412) ccw
  arc A374 (79.442, 13.6372) -> (79.442, 15.6452) centre (79.442, 14.6412) ccw
  arc A375 (79.442, 15.6452) -> (79.442, 13.6372) centre (79.442, 14.6412) ccw
  arc A376 (74.442, 13.6372) -> (74.442, 15.6452) centre (74.442, 14.6412) ccw
  arc A377 (74.442, 15.6452) -> (74.442, 13.6372) centre (74.442, 14.6412) ccw
  arc A378 (74.442, 13.6372) -> (74.442, 15.6452) centre (74.442, 14.6412) ccw
  arc A379 (74.442, 15.6452) -> (74.442, 13.6372) centre (74.442, 14.6412) ccw
  arc A380 (74.442, 8.6372) -> (74.442, 10.6452) centre (74.442, 9.6412) ccw
  arc A381 (74.442, 10.6452) -> (74.442, 8.6372) centre (74.442, 9.6412) ccw
  arc A382 (74.442, 8.6372) -> (74.442, 10.6452) centre (74.442, 9.6412) ccw
  arc A383 (74.442, 10.6452) -> (74.442, 8.6372) centre (74.442, 9.6412) ccw
  point P0 (0, 0)
  constraints: 768 point on circle, 384 centre point, 256 end point